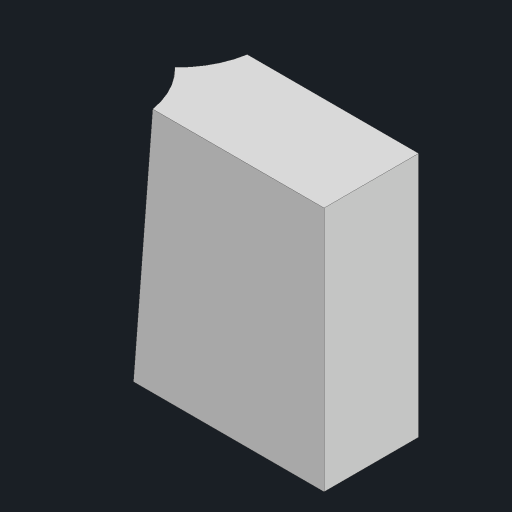
# Autodesk Inventor part: Capper Gate
Saved by Autodesk Inventor 2023.1 (Build 271208000, 208)
## iProperties
Created: 2023-02-21
Part Number: Capper Gate
Material: Generic
Document SubType Name: Modeling
Designer: Jarrett
Density: 1 g/cm^3
Appearance: Default
Author: Jarrett
Autodesk Inventor part; units mm, degrees
ref_plane "YZ Plane" through (0, 0, 0) normal (1, 0, 0) x (0, 1, 0)
ref_plane "XY Plane" through (0, 0, 0) normal (0, 0, 1) x (1, 0, 0)
sketch "Sketch2" plane through (0, 0, 0) normal (0, 1, 0) x (-1, 0, 0)
  circle A0 centre (0, -6.5) radius 6.5 construction
  line L0 (0, -16.9) -> (0, 10.4) projected
  arc A1 (-2.5981, 0) -> (-6.8374, -5) centre (0, -6.5) ccw
  line L1 (-5.5902, -1.5) -> (-27, -1.5)
  line L2 (-5.5902, 0) -> (-5.5902, -1.5)
  line L3 (-5.5902, -1.5) -> (-5.2175, -1.8333) construction
  line L4 (13.2, 0) -> (-33.7, 0) construction
  line L5 (-27, -1.5) -> (-27, -5)
  line L6 (-27, -5) -> (-6.8374, -5)
  line L7 (-7, -6.5) -> (-7, -5) construction
  arc A2 (-6.8374, -5) -> (-7, -6.5) centre (0, -6.5) ccw construction
  line L8 (-7, -5.5) -> (-27, -5.5)
  line L9 (-27, -5.5) -> (-27, -6.5)
  line L10 (-27, -6.5) -> (-7, -6.5)
  line L11 (-13.5902, -1.5) -> (-13.5902, 0)
  line L12 (-9.5902, 0) -> (-9.5902, -1.5)
  line L13 (-27, -1.5) -> (-27, 0)
  arc A3 (-6.8374, 5) -> (-2.5981, 0) centre (0, 6.5) ccw
  line L14 (-5.5902, 1.5) -> (-27, 1.5)
  line L15 (-5.5902, 0) -> (-5.5902, 1.5)
  line L16 (-27, 1.5) -> (-27, 5)
  line L17 (-27, 5) -> (-6.8374, 5)
  line L18 (-13.5902, 1.5) -> (-13.5902, 0)
  line L19 (-9.5902, 0) -> (-9.5902, 1.5)
  line L20 (-27, 1.5) -> (-27, 0)
  point P0 (0, 0)
  point P1 (-2.5981, 0)
  dimension "d0" = 13
  dimension "d2" = 0.5
  dimension "d4" = 0.5
  dimension "d5" = 3
  dimension "d6" = 10
  dimension "d8" = 20
  dimension "d9" = 0.5
  dimension "d11" = 8
  dimension "d27" = 4.4019
  constraints: 38 end point, 12 point on line, 8 point on circle, 7 perpendicular, 7 symmetric about line, 3 centre point, 2 horizontal, 2 line through centre, 2 vertical, 1 collinear, 1 tangent, 1 vertical alignment, 4 other
  measures "d4" distance of L1.start L3.end
  measures "d5" diameter of L1 L4
  measures "d6" diameter of L6 L4
  measures "d8" distance of L9.end L7.start
  measures "d9" distance between parallel lines of L6 L8
  measures "d11" diameter of L2 L12
  measures "d27" distance from line of A1.start L7
ref_plane "Work Plane1" through (0, 26, 0) normal (0, 1, 0) x (-1, 0, 0)
sketch "Sketch3" plane through (0, 26, 0) normal (0, 1, 0) x (-1, 0, 0)
  circle A0 centre (0, -6.5) radius 8.5 construction
  arc A1 (-6.2249, 0) -> (-8.8741, -5) centre (0, -6.5) ccw
  line L0 (-27, -5) -> (-8.8741, -5)
  line L1 (-27, 5) -> (-27, -5)
  line L2 (15.6, 0) -> (-34.1, 0) construction
  arc A2 (-8.8741, 5) -> (-6.2249, 0) centre (0, 6.5) ccw
  line L3 (-8.8741, 5) -> (-27, 5)
  point P0 (0, 0)
  dimension "d16" = 17
  dimension "d17" = 0.5
  constraints: 6 end point, 4 point on circle, 3 centre point, 2 horizontal, 2 symmetric about line, 1 coincident, 1 perpendicular, 1 point on line, 1 other
  measures "d16" diameter of A0
  measures "d17" radial gap between concentric circles of A0 A1
loft "Loft1" add profiles "Sketch3", "Sketch2"
sketch "Sketch5" plane through (6.8374, 0, 5) normal (0, 0, 1) x (1, 0, 0)
  line L0 (-1.2472, 0) -> (0.7895, 26)
  line L1 (2.0367, 26) -> (0, 0) projected
  line L2 (-0.6124, 26) -> (2.0367, 26) projected
  line L3 (-0.6124, 26) -> (-4.2393, 0) projected
  line L4 (-4.2393, 0) -> (0, 0) projected
  line L5 (2.0367, 26) -> (0, 0) projected
  line L6 (2.0367, 26) -> (20.1626, 26) projected
  line L7 (2.0367, 26) -> (0, 0) projected
  line L8 (0, 0) -> (20.1626, 0) projected
  line L9 (20.1626, 26) -> (20.1626, 0) projected
  circle A0 centre (5.1232, 15.876) radius 4.6543
  line L10 (8.727, 18.8214) -> (19.6547, 23.4226)
  point P0 (-6.8374, 0)
  constraints: 4 end point, 1 parallel, 1 point on line, 3 other
body "Solid2"
